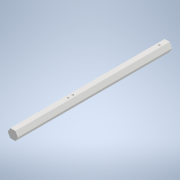
# Autodesk Inventor part: eje4_n
Saved by Autodesk Inventor 2022 (Build 260153000, 153)
## iProperties
Created: 2022-03-11
Part Number: eje4_n
Material: Generic
Document SubType Name: Modeling
Designer: katha
Density: 1 g/cm^3
Appearance: Default
Author: katha
Autodesk Inventor part; units mm, degrees
ref_plane "YZ Plane" through (0, 0, 0) normal (1, 0, 0) x (0, 1, 0)
ref_plane "XZ Plane" through (0, 0, 0) normal (0, 1, 0) x (-1, 0, 0)
ref_plane "XY Plane" through (0, 0, 0) normal (0, 0, 1) x (1, 0, 0)
sketch "Sketch1" plane through (0, 0, 0) normal (0, 0, 1) x (1, 0, 0)
  circle A0 centre (0, 0) radius 7.5 projected
  line L0 (-1.7809, 3.0847) -> (1.7809, 3.0847) projected
  line L1 (0, 0) -> (3.1, 0) construction
  line L2 (0, 0) -> (1.55, 2.6847) construction
  line L3 (0, 0) -> (-1.55, 2.6847) construction
  line L4 (0, 0) -> (-3.1, 0) construction
  line L5 (0, 0) -> (-1.55, -2.6847) construction
  line L6 (0, 0) -> (1.55, -2.6847) construction
  line L7 (-1.55, 2.6847) -> (1.55, 2.6847)
  line L8 (1.55, 2.6847) -> (3.1, 0)
  line L9 (3.1, 0) -> (1.55, -2.6847)
  line L10 (1.55, -2.6847) -> (-1.55, -2.6847)
  line L11 (-1.55, -2.6847) -> (-3.1, 0)
  line L12 (-3.1, 0) -> (-1.55, 2.6847)
  dimension "d0" = 3.1
  dimension "d3" = 360
  constraints: 24 end point, 3 parallel, 2 coincident, 2 horizontal, 17 other
  measures "d0" distance of L1.start L1.end
extrude "Extrusion1" add sketch "Sketch1" against normal blind 95 contours L7 L8 L9 L10 L11 L12
sketch "Sketch2" plane through (-1.55, 2.6847, 0) normal (0, 1, 0) x (1, 0, 0)
  line L0 (0, 0) -> (0, 95) projected
  line L1 (3.1, 0) -> (3.1, 95) projected
  circle A0 centre (1.55, 33.9) radius 0.65
  circle A1 centre (1.55, 36.9) radius 0.65
  line L2 (3.1, 0) -> (0, 0) projected
  circle A2 centre (1.5626, 33.9) radius 0.65 projected
  circle A3 centre (1.55, 90) radius 0.65
  line L3 (0, 95) -> (3.1, 95) projected
  point P0 (1.55, 0)
  point P1 (1.55, 0)
  point P2 (1.55, 0)
  point P3 (1.5563, 34.55)
  point P4 (1.5563, 33.25)
  dimension "d7" = 1.3
  dimension "d8" = 3
  dimension "d9" = 33.9
  dimension "d10" = 5
  constraints: 3 centre point, 3 vertical alignment, 2 equal radius, 2 midpoint
  measures "d7" diameter of A0
  measures "d8" distance of A1.centre A0.centre
  measures "d9" distance from line of L2 A0.centre
  measures "d10" distance from line of A3.centre L3
extrude "Extrusion2" cut sketch "Sketch2" against normal blind 10 contours A0 A2 | A1 | A3 picked at (1.3449, 33.9)
body "Solid1"
